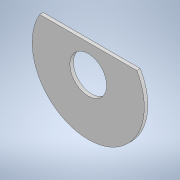
# Autodesk Inventor part: 68. Пластина упорная
Saved by Autodesk Inventor 2021 (Build 250183000, 183)
## iProperties
Created: 2021-03-11
Part Number: 68. Пластина упорная
Material: Типовые
Document SubType Name: Modeling
Designer: Данил
Density: 1 g/cm^3
Appearance: По умолчанию
Author: Данил
Autodesk Inventor part; units mm, degrees
ref_plane "YZ Plane" through (0, 0, 0) normal (1, 0, 0) x (0, 1, 0)
ref_plane "XZ Plane" through (0, 0, 0) normal (0, 1, 0) x (-1, 0, 0)
ref_plane "XY Plane" through (0, 0, 0) normal (0, 0, 1) x (1, 0, 0)
sketch "Эскиз1" plane through (0, 0, 0) normal (0, 0, 1) x (1, 0, 0)
  circle A0 centre (0, 0) radius 5.25
  line L0 (0, 0) -> (0, 8) construction
  line L1 (-13.8564, 8) -> (13.8564, 8)
  arc A1 (-13.8564, 8) -> (13.8564, 8) centre (0, 0) ccw
  dimension "d0" = 10.5
  dimension "d1" = 8
  dimension "d2" = 16
  constraints: 5 coincident, 4 end point, 2 centre point, 2 point on circle, 1 horizontal, 1 horizontal alignment, 1 midpoint, 1 vertical
  measures "d0" diameter of A0
  measures "d1" distance of L0.end L0.start
  measures "d2" radius of A1
extrude "Выдавливание1" add sketch "Эскиз1" along normal mid plane 1
